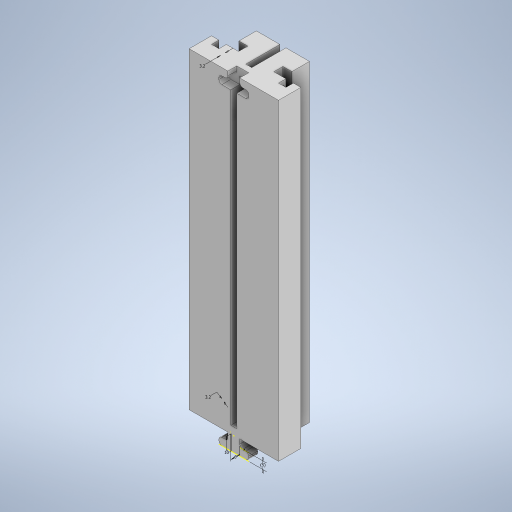
# Autodesk Inventor part: 밑판
Saved by Autodesk Inventor 2023 (Build 270158000, 158)
## iProperties
Created: 2023-04-28
Part Number: 밑판
Material: 일반
Document SubType Name: Modeling
Designer: rlatk
Density: 1 g/cm^3
Appearance: 기본값
Author: rlatk
Autodesk Inventor part; units mm, degrees
ref_plane "YZ Plane" through (0, 0, 0) normal (1, 0, 0) x (0, 1, 0)
ref_plane "XZ Plane" through (0, 0, 0) normal (0, 1, 0) x (-1, 0, 0)
ref_plane "XY Plane" through (0, 0, 0) normal (0, 0, 1) x (1, 0, 0)
sketch "스케치1" plane through (0, 0, 0) normal (0, 1, 0) x (-1, 0, 0)
  line L0 (-17.8, -18) -> (-17.8, -6.2)
  line L1 (-11.8155, 0) -> (11.8052, 0)
  line L2 (17.8, -6.2) -> (17.8, -17.9333)
  line L3 (11.8052, 0) -> (11.7948, -6.2)
  line L4 (11.7948, -6.2) -> (17.8, -6.2)
  line L5 (-11.8155, 0) -> (-11.7845, -6.2)
  line L6 (-11.7845, -6.2) -> (-17.8, -6.2)
  line L7 (-30, 0) -> (-30, 15)
  line L8 (-30, 15) -> (30, 15)
  line L9 (30, 15) -> (30, 0)
  line L10 (-2, -18) -> (-2, 5)
  line L11 (-2, 5) -> (2, 5)
  line L12 (2, 5) -> (2, -17.9333)
  line L13 (17.8, -17.9333) -> (2, -17.9333)
  line L14 (-2, -18) -> (-17.8, -18)
  line L15 (20, 0) -> (20, 5)
  line L16 (20, 5) -> (25, 5)
  line L17 (25, 5) -> (25, 0)
  line L18 (-25, 0) -> (-25, 5)
  line L19 (-25, 5) -> (-20, 5)
  line L20 (-20, 5) -> (-20, 0)
  line L21 (30, 0) -> (25, 0)
  line L22 (20, 0) -> (-20, 0)
  line L23 (-25, 0) -> (-30, 0)
  point P0 (0, 0)
  point P1 (0, 0)
  point P2 (-14.7922, -6.2)
  point P3 (-0.0051, 0)
  point P4 (0, 5)
  point P5 (25, 2.5)
  point P6 (-25, 2.5)
  point P7 (11.8052, 0)
  point P8 (-11.8155, 0)
  point P9 (17.8, -12.0667)
  point P10 (0, 0)
  point P11 (14.7974, -6.2)
  point P12 (11.8, -3.1)
  point P13 (-11.8, -3.1)
  dimension "d5" = 60
  dimension "d11" = 4
  dimension "d17" = 5
  dimension "d18" = 5
  dimension "d25" = 15.8
  dimension "d26" = 15.8
  dimension "d27" = 2
  dimension "d28" = 2
  dimension "d29" = 6.2
  dimension "d30" = 6.2
  dimension "d31" = 9.8
  dimension "d32" = 9.8
  constraints: 48 end point, 10 midpoint, 10 parallel, 5 horizontal, 5 perpendicular, 3 point on line, 1 coincident
  measures "d5" distance of L7.end L8.end
  measures "d11" distance of L10.end L11.end
  measures "d17" distance from line of L9 point (25, 2.5)
  measures "d18" distance from line of L7 point (-25, 2.5)
  measures "d25" distance between parallel lines of L10 L0
  measures "d26" distance from line of point (17.8, -12.067) L12
  measures "d27" distance from line of point (0, 0) L10
  measures "d28" distance from line of L12 point (0, 0)
  measures "d29" distance between parallel lines of L6 L22
  measures "d30" distance from line of point (14.797, -6.2) L22
  measures "d31" distance from line of L12 point (11.8, -3.1)
  measures "d32" distance from line of L10 point (-11.8, -3.1)
extrude "돌출1" add sketch "스케치1" along normal blind 210 contours L0 L6 L5 L1 L10 L14 | L1 L22 L20 L19 L18 L23 L7 L8 L9 L21 L17 L16 L15 L12 L11 L10 | L1 L3 L4 L2 L13 L12
sketch "스케치2" plane through (-30, 0, 15) normal (0, 0, 1) x (1, 0, 0)
  line L0 (28, 0) -> (28, 210) projected
  line L1 (32, 0) -> (32, 210) projected
  line L2 (28, 210) -> (32, 210)
  line L3 (32, 210) -> (32, 0)
  line L4 (32, 0) -> (28, 0)
  line L5 (28, 0) -> (28, 210)
  line L6 (28, 5) -> (32, 5)
  line L7 (28, 205) -> (32, 205)
  point P0 (30, 0)
  point P1 (30, 0)
  point P2 (30, 5)
  point P3 (30, 210)
  point P4 (30, 205)
  dimension "d21" = 5
  dimension "d22" = 5
  constraints: 12 end point, 5 point on line, 4 midpoint, 3 perpendicular, 2 parallel, 1 horizontal
  measures "d21" distance of point (30, 0) point (30, 5)
  measures "d22" distance of point (30, 210) point (30, 205)
extrude "돌출2" cut sketch "스케치2" against normal blind 10 contours L0 L7 L1 L6
sketch "스케치4" plane through (-2, 0, 5) normal (1, 0, 0) x (0, 0, -1)
  line L0 (-10, 0) -> (-4, 0)
  line L1 (-4, 0) -> (-4, -10)
  line L2 (-4, -10) -> (-10, -10)
  line L3 (-10, -10) -> (-10, 0)
  line L4 (-4, -5) -> (-10, -5)
  point P0 (5, 0)
  dimension "d33" = 6
  dimension "d34" = 10
  constraints: 10 end point, 2 midpoint, 2 parallel, 1 horizontal, 1 perpendicular
  measures "d33" distance of L1.end L2.end
  measures "d34" distance between parallel lines of L2 L0
extrude "돌출3" add sketch "스케치4" along normal blind 6 and the other way blind 2
extrude "돌출4" add sketch "스케치4" along normal blind 12 and the other way blind 8 contours L4 L1 L2 L3
sketch "스케치5" plane through (-30, 210, 15) normal (0, 0, 1) x (1, 0, 0)
  line L0 (0, 0) -> (60, 0) projected
  line L1 (34, 0) -> (26, 0)
  line L2 (26, 0) -> (26, -9.9)
  line L3 (26, -9.9) -> (34, -9.9)
  line L4 (34, -9.9) -> (34, 0)
  line L5 (34, -4.95) -> (26, -4.95)
  line L6 (40.05, -4.8) -> (19.95, -4.8)
  line L7 (19.95, -4.8) -> (19.95, -9.9)
  line L8 (19.95, -9.9) -> (40.05, -9.9)
  line L9 (40.05, -9.9) -> (40.05, -4.8)
  point P0 (30, -210)
  point P1 (30, 0)
  point P2 (30, -9.9)
  point P3 (34, -4.8)
  point P4 (26, 0)
  point P5 (26, -4.8)
  dimension "d43" = 8
  dimension "d44" = 9.9
  dimension "d45" = 20.1
  dimension "d48" = 5.1
  constraints: 18 end point, 6 midpoint, 4 parallel, 2 horizontal, 2 perpendicular, 1 point on line
  measures "d43" distance of L3.end L2.end
  measures "d44" distance of L2.end L1.end
  measures "d45" distance of L8.end L7.end
  measures "d48" distance between parallel lines of L6 L8
extrude "돌출5" cut sketch "스케치5" against normal blind 6
sketch "스케치6" plane through (-30, 0, 15) normal (0, 0, 1) x (1, 0, 0)
  line L0 (34, -5) -> (40, -5) projected
  line L1 (20, -10) -> (40, -10) projected
  point P0 (30, 0)
  point P1 (37, -5)
  dimension "d49" = 5
  constraints: 1 midpoint
  measures "d49" distance from line of point (37, -5) L1
fillet "모깎기1" radius 2 4 edges at (10, -10, 12) (10, -5, 12) (-10, -10, 12) (-10, -5, 12)
fillet "모깎기2" radius 2 8 edges at (-10.05, 205.2, 12) (10.05, 205.2, 12) (-10.05, 200.1, 12) (10.05, 200.1, 12) (-4, 205.2, 12) (4, 205.2, 12) (-4, -5, 12) (4, -5, 12)
sketch "스케치7" plane through (-20, 0, 0) normal (-1, 0, 0) x (0, 0, 1)
  circle A0 centre (2.4189, 205.5275) radius 1.6
  circle A1 centre (2.4189, 4.2737) radius 1.6
  point P0 (0, 0)
  dimension "d52" = 3.2
  dimension "d53" = 3.2
  constraints: 2 centre point
  measures "d52" diameter of A0
  measures "d53" diameter of A1
extrude "돌출6" cut sketch "스케치7" against normal blind 41.75 contours A1
extrude "돌출7" cut sketch "스케치7" against normal blind 41.75 contours A0
sketch "스케치8" plane through (4, 0, 9) normal (0, 0, -1) x (-1, 0, 0)
  point P0 (4, 0)
